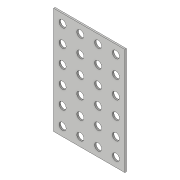
# Autodesk Inventor part: Base_modulos
Saved by Autodesk Inventor 2017 (Build 210142000, 142)
## iProperties
Created: 2017-06-21
Part Number: Base_modulos
Material: Generic
Document SubType Name: Modeling
Designer: Butri
Density: 1 g/cm^3
Appearance: Default
Author: Butri
Autodesk Inventor part; units mm, degrees
ref_plane "YZ Plane" through (0, 0, 0) normal (1, 0, 0) x (0, 1, 0)
ref_plane "XZ Plane" through (0, 0, 0) normal (0, 1, 0) x (-1, 0, 0)
ref_plane "XY Plane" through (0, 0, 0) normal (0, 0, 1) x (1, 0, 0)
sketch "Sketch1" plane through (0, 0, 0) normal (0, 1, 0) x (-1, 0, 0)
  line L0 (140, 210) -> (-140, 210)
  line L1 (-140, 210) -> (-140, -210)
  line L2 (-140, -210) -> (140, -210)
  line L3 (140, -210) -> (140, 210)
  line L4 (140, 210) -> (-140, -210) construction
  line L5 (-140, 210) -> (140, -210) construction
  point P0 (0, 0)
  dimension "d0" = 280
  dimension "d1" = 420
  constraints: 12 end point, 2 midpoint, 2 parallel, 1 horizontal, 1 perpendicular
  measures "d0" distance of L2.end L1.end
  measures "d1" distance of L1.end L0.end
extrude "Extrusion1" add sketch "Sketch1" along normal blind 6
sketch "Sketch2" plane through (0, 6, 0) normal (0, 1, 0) x (1, 0, 0)
  circle A0 centre (105, -175) radius 14
  line L0 (-140, -210) -> (140, -210) projected
  line L1 (140, -210) -> (140, 210) projected
  point P0 (0, 0)
  dimension "d4" = 28
  dimension "d5" = 35
  dimension "d6" = 35
  constraints: 1 centre point
  measures "d4" diameter of A0
  measures "d5" distance from line of L0 A0.centre
  measures "d6" distance from line of L1 A0.centre
extrude "Extrusion2" cut sketch "Sketch2" against normal blind 6
sketch "Sketch3" plane through (0, 6, 0) normal (0, 1, 0) x (1, 0, 0)
  circle A0 centre (135, -205) radius 1.75
  line L0 (-140, -210) -> (140, -210) projected
  line L1 (140, -210) -> (140, 210) projected
  circle A1 centre (75.5, -205) radius 1.75
  circle A2 centre (135, -145.5) radius 1.75
  circle A3 centre (75.5, -145.5) radius 1.75
  point P0 (0, 0)
  dimension "d15" = 3.5
  dimension "d16" = 5
  dimension "d17" = 5
  dimension "d18" = 3.5
  dimension "d19" = 5
  dimension "d20" = 59.5
  dimension "d21" = 3.5
  dimension "d22" = 5
  dimension "d23" = 59.5
  dimension "d24" = 3.5
  dimension "d25" = 59.5
  dimension "d26" = 59.5
  constraints: 4 centre point
  measures "d15" diameter of A0
  measures "d16" distance from line of L0 A0.centre
  measures "d17" distance from line of L1 A0.centre
  measures "d18" diameter of A1
  measures "d19" distance from line of L0 A1.centre
  measures "d20" distance of A1.centre A0.centre
  measures "d21" diameter of A2
  measures "d22" distance from line of L1 A2.centre
  measures "d23" distance of A0.centre A2.centre
  measures "d24" diameter of A3
  measures "d25" distance of A2.centre A3.centre
  measures "d26" distance of A1.centre A3.centre
pattern_linear "Rectangular Pattern1" count 6 spacing 70 along (0, 0, -1) count 4 spacing 70 along (-1, 0, 0) of "Extrusion2"
equation "\"d17\" = d16"
equation "\"d19\" = d16"
equation "\"d22\" = d16"
equation "\"d23\" = d20"
equation "\"d25\" = d20"
equation "\"d26\" = d20"
body "Solid1"
